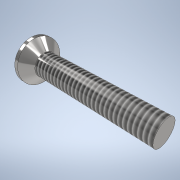
# Autodesk Inventor part: Болт М3х15
Saved by Autodesk Inventor 2021.1 (Build 251245010, 245A)
## iProperties
Created: 2026-05-18
Part Number: Болт М3х15
Material: Типовые
Document SubType Name: Modeling
Designer: Андрей Тарасов
Density: 1 g/cm^3
Appearance: По умолчанию
Author: Андрей Тарасов
Autodesk Inventor part; units mm, degrees
ref_plane "YZ Plane" through (0, 0, 0) normal (1, 0, 0) x (0, 1, 0)
ref_plane "XZ Plane" through (0, 0, 0) normal (0, 1, 0) x (-1, 0, 0)
ref_plane "XY Plane" through (0, 0, 0) normal (0, 0, 1) x (1, 0, 0)
sketch "Эскиз4" plane through (0, 0, 0) normal (0, 0, 1) x (1, 0, 0)
  line L0 (0, 0) -> (0, 2.75)
  line L1 (1.6, 1.45) -> (16, 1.45)
  line L2 (16, 1.45) -> (16, 0)
  line L3 (16, 0) -> (0, 0)
  line L4 (0, 2.75) -> (0.5, 2.75)
  line L5 (0.5, 2.75) -> (1.6, 1.45)
  dimension "d14" = 16
  dimension "d15" = 1.45
  dimension "d17" = 2.75
  dimension "d18" = 0.5
  dimension "d19" = 1.6
  constraints: 12 end point, 3 perpendicular, 1 horizontal, 1 vertical
  measures "d14" distance between parallel lines of L2 L0
  measures "d15" distance between parallel lines of L3 L1
  measures "d17" distance of L0.start L0.end
  measures "d18" distance of L0.end L4.end
  measures "d19" distance from line of L1.start L0
revolve "Вращение1" add sketch "Эскиз4" angle 360 about axis through (16, 0, 0) along (-1, 0, 0)
thread "Резьба2" size "M3x0.5" class "6g" standard "ANSI Metric M Profile" full length
sketch "Эскиз5" plane through (0, 0, 0) normal (-1, 0, 0) x (0, 0, 1)
  line L0 (0.5, -2) -> (-0.5, -2)
  line L1 (-0.5, -2) -> (-0.5, 2)
  line L2 (-0.5, 2) -> (0.5, 2)
  line L3 (0.5, 2) -> (0.5, -2)
  line L4 (0.5, -2) -> (-0.5, 2) construction
  line L5 (-0.5, -2) -> (0.5, 2) construction
  line L6 (-2, -0.5) -> (2, -0.5)
  line L7 (2, -0.5) -> (2, 0.5)
  line L8 (2, 0.5) -> (-2, 0.5)
  line L9 (-2, 0.5) -> (-2, -0.5)
  circle A0 centre (0, 0) radius 2.75 projected
  line L10 (-2, -0.5) -> (2, 0.5) construction
  line L11 (2, -0.5) -> (-2, 0.5) construction
  point P0 (-0.5, 0.5)
  point P1 (-0.5, -0.5)
  point P2 (0.5, -0.5)
  point P3 (0.5, 0.5)
  dimension "d23" = 1
  dimension "d24" = 4
  constraints: 24 end point, 4 midpoint, 4 parallel, 4 perpendicular, 2 horizontal
  measures "d23" distance of L6.end L7.end
  measures "d24" distance of L6.start L6.end
extrude "Выдавливание4" cut sketch "Эскиз5" against normal blind 1 contours L0 L1 L6 L3 | L6 L1 L8 L3 | L3 L8 L7 L6 | L6 L9 L8 L1 | L8 L1 L2 L3
